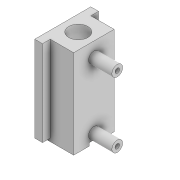
# Autodesk Inventor part: Tube_outerhole_template_p1
Saved by Autodesk Inventor 2022 (Build 260153000, 153)
## iProperties
Created: 2022-05-02
Part Number: Tube_outerhole_template_p1
Material: Generic
Document SubType Name: Modeling
Designer: dell
Density: 1 g/cm^3
Appearance: Default
Author: dell
Autodesk Inventor part; units mm, degrees
ref_plane "YZ Plane" through (0, 0, 0) normal (1, 0, 0) x (0, 1, 0)
ref_plane "XZ Plane" through (0, 0, 0) normal (0, 1, 0) x (-1, 0, 0)
ref_plane "XY Plane" through (0, 0, 0) normal (0, 0, 1) x (1, 0, 0)
sketch "Sketch1" plane through (0, 0, 0) normal (0, 1, 0) x (-1, 0, 0)
  circle A0 centre (0, 0) radius 6.15
  line L0 (10, 13) -> (-10, 13)
  line L1 (-10, 13) -> (-10, -13)
  line L2 (-10, -13) -> (10, -13)
  line L3 (10, -13) -> (10, 13)
  dimension "d0" = 12.3
  dimension "d1" = 10
  dimension "d2" = 10
  dimension "d3" = 13
  dimension "d4" = 13
  constraints: 8 end point, 2 parallel, 1 centre point, 1 coincident, 1 horizontal, 1 perpendicular
  measures "d0" diameter of A0
  measures "d1" distance from line of point (0, 0) L1
  measures "d2" distance from line of point (0, 0) L3
  measures "d3" distance from line of point (0, 0) L2
  measures "d4" distance from line of point (0, 0) L0
extrude "Extrusion1" add sketch "Sketch1" along normal blind 55
sketch "Sketch2" plane through (10, 0, 13) normal (1, 0, 0) x (0, 0, -1)
  circle A0 centre (13, 4) radius 1.45
  line L0 (0, 0) -> (26, 0) projected
  circle A1 centre (13, 46) radius 1.45
  line L1 (0, 0) -> (0, 55) projected
  point P0 (13, 0)
  dimension "d7" = 2.9
  dimension "d8" = 4
  dimension "d9" = 2.9
  dimension "d10" = 46
  dimension "d11" = 13
  dimension "d12" = 13
  constraints: 2 centre point
  measures "d7" diameter of A0
  measures "d8" distance from line of L0 A0.centre
  measures "d9" diameter of A1
  measures "d10" distance from line of L0 A1.centre
  measures "d11" distance from line of L1 A0.centre
  measures "d12" distance from line of L1 A1.centre
extrude "Extrusion2" cut sketch "Sketch2" against normal blind 55
sketch "Sketch3" plane through (10, 0, 13) normal (1, 0, 0) x (0, 0, -1)
  circle A0 centre (13, 4) radius 1.45 projected
  circle A1 centre (13, 46) radius 1.45 projected
  line L0 (0, 0) -> (26, 0) projected
  line L1 (26, 0) -> (26, 55) projected
  line L2 (0, 55) -> (26, 55) projected
  line L3 (0, 0) -> (0, 55) projected
  circle A2 centre (13, 46) radius 3.45
  circle A3 centre (13, 4) radius 3.45
  circle A4 centre (4, 46) radius 1.6
  circle A5 centre (22, 46) radius 1.6
  circle A6 centre (4, 4) radius 1.6
  circle A7 centre (22, 4) radius 1.6
  point P0 (13, 0)
  dimension "d15" = 2
  dimension "d16" = 2
  dimension "d19" = 3.2
  dimension "d20" = 3.2
  dimension "d21" = 3.2
  dimension "d22" = 3.2
  dimension "d23" = 4
  dimension "d24" = 4
  dimension "d25" = 4
  dimension "d26" = 4
  constraints: 6 centre point
  measures "d15" radial gap between concentric circles of A1 A2
  measures "d16" radial gap between concentric circles of A0 A3
  measures "d19" diameter of A4
  measures "d20" diameter of A5
  measures "d21" diameter of A6
  measures "d22" diameter of A7
  measures "d23" distance from line of L3 A6.centre
  measures "d24" distance from line of L1 A7.centre
  measures "d25" distance from line of L3 A4.centre
  measures "d26" distance from line of L1 A5.centre
extrude "Extrusion3" add sketch "Sketch3" along normal blind 15 contours A2 | A3
sketch "Sketch6" plane through (-10, 0, 13) normal (0, 0, 1) x (1, 0, 0)
  line L0 (20, 55) -> (0, 55) projected
  line L1 (20, 0) -> (0, 0) projected
  line L2 (0, 55) -> (5, 55)
  line L3 (5, 55) -> (5, 0)
  line L4 (5, 0) -> (0, 0)
  line L5 (0, 0) -> (0, 55)
  point P0 (10, 0)
  point P1 (5, 55)
  dimension "d31" = 5
  constraints: 8 end point, 2 parallel, 1 horizontal, 1 perpendicular, 1 point on line
  measures "d31" distance between parallel lines of L5 L3
extrude "Extrusion6" add sketch "Sketch6" along normal blind 5
sketch "Sketch7" plane through (10, 0, -13) normal (0, 0, -1) x (-1, 0, 0)
  line L0 (20, 55) -> (20, 0) projected
  line L1 (20, 0) -> (15, 0) projected
  line L2 (20, 55) -> (15, 55)
  line L3 (15, 55) -> (15, 0)
  line L4 (15, 0) -> (20, 0)
  line L5 (20, 0) -> (20, 55)
  point P0 (10, 0)
  dimension "d34" = 5
  constraints: 8 end point, 2 parallel, 1 horizontal, 1 perpendicular, 1 point on line
  measures "d34" distance between parallel lines of L0 L3
extrude "Extrusion7" add sketch "Sketch7" along normal blind 5
sketch "Sketch8" plane through (0, 0, 0) normal (0, -1, 0) x (1, 0, 0)
  line L0 (10, 13) -> (10, -13) projected
  line L1 (-10, 18) -> (-10, -18) projected
  line L2 (10, 13) -> (-10, 13)
  line L3 (-10, 13) -> (-10, 3)
  line L4 (-10, 3) -> (10, 3)
  line L5 (10, 3) -> (10, 13)
  line L6 (10, -13) -> (-5, -13) projected
  line L7 (10, -13) -> (-10, -13)
  line L8 (-10, -13) -> (-10, -3)
  line L9 (-10, -3) -> (10, -3)
  line L10 (10, -3) -> (10, -13)
  point P0 (0, 0)
  point P1 (10, -3)
  point P2 (-10, -3)
  dimension "d37" = 10
  dimension "d38" = 10
  constraints: 16 end point, 4 parallel, 2 horizontal, 2 perpendicular, 2 point on line
  measures "d37" distance between parallel lines of L6 L9
  measures "d38" distance between parallel lines of L2 L4
extrude "Extrusion8" add sketch "Sketch8" along normal blind 2 contours L0 L4 L1 L2 | L0 L6 L7 L1 L9
body "Solid1"
